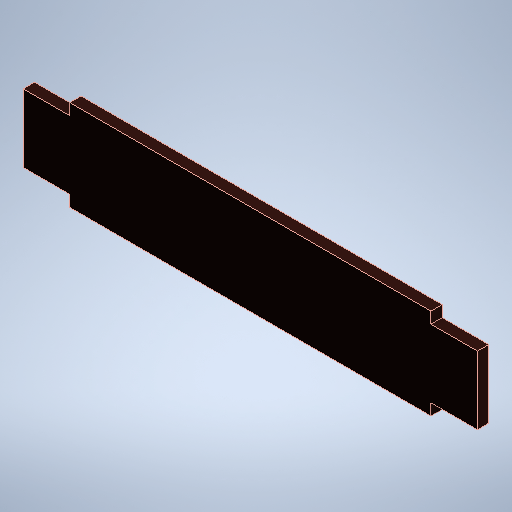
# Autodesk Inventor part: Base Leg V1
Saved by Autodesk Inventor 2025.4 (Build 294407000, 407)
## iProperties
Created: 2026-03-23
Part Number: Base Leg V1
Material: Generic
Document SubType Name: Sheet Metal
Designer: lenovo
Density: 1 g/cm^3
Sheet Metal Rule: Default_mm
Appearance: Default(1)
Author: lenovo
Autodesk Inventor part; units mm, degrees
ref_plane "YZ Plane" through (0, 0, 0) normal (1, 0, 0) x (0, 1, 0)
ref_plane "XZ Plane" through (0, 0, 0) normal (0, 1, 0) x (-1, 0, 0)
ref_plane "XY Plane" through (0, 0, 0) normal (0, 0, 1) x (1, 0, 0)
sketch "Sketch1" plane through (0, 0, 0) normal (0, 0, 1) x (1, 0, 0)
  line L0 (-100, -15) -> (100, -15)
  line L1 (100, -15) -> (100, 15)
  line L2 (100, 15) -> (-100, 15)
  line L3 (-100, 15) -> (-100, -15)
  line L4 (-100, -15) -> (100, 15) construction
  line L5 (100, -15) -> (-100, 15) construction
  line L6 (-79.5, 20) -> (79.5, 20)
  line L7 (79.5, 20) -> (79.5, 15)
  line L8 (79.5, 15) -> (-79.5, 15)
  line L9 (-79.5, 15) -> (-79.5, 20)
  line L10 (-79.5, 20) -> (79.5, 15) construction
  line L11 (79.5, 20) -> (-79.5, 15) construction
  line L12 (-100, 0) -> (100, 0)
  line L13 (-79.5, -20) -> (79.5, -20)
  line L14 (79.5, -20) -> (79.5, -15)
  line L15 (79.5, -15) -> (-79.5, -15)
  line L16 (-79.5, -15) -> (-79.5, -20)
  line L17 (-79.5, -20) -> (79.5, -15) construction
  line L18 (79.5, -20) -> (-79.5, -15) construction
  point P0 (0, 0)
  point P1 (0, 17.5)
  point P2 (0, 15)
  point P3 (0, -17.5)
  point P4 (0, -15)
  dimension "d0" = 5
  dimension "d1" = 30
  dimension "d2" = 200
  dimension "d3" = 159
  measures "d0" distance of L8.end L6.start
  measures "d1" distance of L2.end L0.start
  measures "d2" distance of L0.start L0.end
  measures "d3" distance of L6.start L6.end
extrude "Plate1" add sketch "Sketch1" along normal blind 5
equation "\"d4\" = Thickness"
equation "\"BendRadius\" = Thickness"
equation "\"BendReliefWidth\" = Thickness"
equation "\"BendReliefDepth\" = 0.5 * Thickness"
equation "\"TransitionRadius\" = BendRadius"
equation "\"JacobiRadiusSize\" = BendRadius"
equation "\"GapSize\" = Thickness"
equation "\"Thickness\" = 5"
body "Solid1"
